Autodesk Fusion 360 part; units mm, degrees
(part 3 of 3)
sketch "bottom_d_plate" plane through (0, 0, 0) normal (0, 1, 0) x (1, 0, 0)
  arc A0 (69.1916, -25.8629) -> (70.1916, -26.8607) centre (70.1916, -25.8607) ccw
  line L0 (69.6545, -38.7668) -> (79.5366, -38.7668)
  circle A1 centre (53.7342, -72.0705) radius 1.7
  arc A2 (-18.6223, 40.5765) -> (-23.9656, 38.9319) centre (-18.6231, 31.0765) ccw
  line L1 (-55.4675, 17.5074) -> (-23.9656, 38.9319)
  arc A3 (53.2919, -80.5601) -> (61.3893, -75.8117) centre (53.1625, -71.0609) ccw
  line L2 (20.548, 40.3463) -> (46.7337, 34.5163)
  line L3 (69.0702, 28.465) -> (69.0699, 28.4264)
  arc A4 (80.543, 19.3715) -> (73.1075, 28.6444) centre (71.043, 19.3715) ccw
  line L4 (25.063, -80.0083) -> (-19.071, -59.5488)
  arc A5 (25.063, -80.0083) -> (29.1879, -80.8885) centre (29.0585, -71.3894) ccw
  line L5 (53.2919, -80.5601) -> (29.1879, -80.8885)
  line L6 (79.2698, -44.8485) -> (61.3893, -75.8117)
  arc A6 (79.2698, -44.8485) -> (80.5358, -39.7279) centre (71.043, -40.0977) ccw
  arc A7 (50.4596, -69.0135) -> (51.8256, -68.6475) centre (50.9596, -68.1475) ccw
  line L7 (-18.6223, 40.5765) -> (18.4843, 40.5734)
  circle A8 centre (-51.125, -50.075) radius 1.7
  circle A9 centre (72.1849, -22.8607) radius 1.7
  arc A10 (20.548, 40.3463) -> (18.4843, 40.5734) centre (18.4835, 31.0734) ccw
  line L8 (-50.125, -58.575) -> (-23.4871, -58.575)
  arc A11 (-59.625, -49.075) -> (-50.125, -58.575) centre (-50.125, -49.075) ccw
  line L9 (69.1916, -25.8629) -> (69.0702, 28.465)
  line L10 (80.543, 19.3715) -> (80.543, -25.8607)
  line L11 (73.1075, 28.6444) -> (70.2865, 29.3961)
  line L12 (-59.625, -49.075) -> (-59.625, 9.652)
  line L13 (69.0702, 28.465) -> (69.1309, 1.3011)
  arc A12 (70.3273, 29.3852) -> (69.0699, 28.4264) centre (70.0698, 28.4189) ccw
  arc A13 (-19.071, -59.5488) -> (-23.4871, -58.575) centre (-23.4871, -69.075) ccw
  circle A14 centre (72.1849, 20.1393) radius 1.7
  line L14 (70.2865, 29.3961) -> (70.3273, 29.3852)
  line L15 (46.7337, 34.5163) -> (46.8423, 34.4921)
  arc A15 (-55.4675, 17.5074) -> (-59.625, 9.652) centre (-50.125, 9.652) ccw
  circle A16 centre (-51.125, 10.1813) radius 1.7
  line L16 (80.543, -40.0977) -> (80.543, -39.4973)
  line L17 (70.1916, -26.8607) -> (79.543, -26.8607)
  arc A17 (80.5358, -39.7279) -> (79.5366, -38.7668) centre (79.5366, -39.7668) ccw
  arc A18 (79.543, -26.8607) -> (80.543, -25.8607) centre (79.543, -25.8607) ccw
  arc A19 (52.2962, -60.5122) -> (53.6622, -60.1462) centre (52.7962, -59.6462) ccw
  line L18 (13.286, -51.6) -> (1.286, -51.6)
  line L19 (36.0873, -42.1814) -> (24.4962, -39.0756)
  line L20 (33.6886, -54.9973) -> (36.7944, -43.4062)
  line L21 (45.1, -3) -> (45.1, -15)
  arc A20 (44.1, 17.05) -> (45.1, 16.05) centre (44.1, 16.05) cw
  circle A21 centre (-18.9309, 32.0765) radius 1.7
  line L22 (45.1, 16.05) -> (45.1, 4.05)
  line L23 (-32.1, 8.05) -> (-44.1, 8.05)
  arc A22 (-26.05, 19.05) -> (-25.05, 20.05) centre (-25.05, 19.05) cw
  line L24 (-12.05, -19.06) -> (-12.05, -31.06)
  circle A23 centre (43.1794, 26.5995) radius 1.7
  line L25 (7, 25.05) -> (7, 13.05)
  arc A24 (-31.1, 7.05) -> (-32.1, 8.05) centre (-32.1, 7.05) ccw
  line L26 (13.05, 0.5) -> (25.05, 0.5)
  arc A25 (6, 26.05) -> (7, 25.05) centre (6, 25.05) cw
  line L27 (6, 12.05) -> (-6, 12.05)
  line L28 (-44.1, -5.95) -> (-32.1, -5.95)
  line L29 (-32.1, -44.05) -> (-44.1, -44.05)
  arc A26 (-45.1, -31.05) -> (-44.1, -30.05) centre (-44.1, -31.05) cw
  line L30 (26.05, 18.55) -> (26.05, 6.55)
  arc A27 (-7, 6) -> (-6, 7) centre (-6, 6) cw
  line L31 (-31.1, -31.05) -> (-31.1, -43.05)
  arc A28 (6, 7) -> (7, 6) centre (6, 6) cw
  arc A29 (26.05, -12.5) -> (25.05, -13.5) centre (25.05, -12.5) cw
  arc A30 (-12.05, -31.06) -> (-13.05, -32.06) centre (-13.05, -31.06) cw
  circle A31 centre (-18.212, -50.5781) radius 1.7
  line L32 (-32.1, -25) -> (-44.1, -25)
  arc A32 (-12.05, -12) -> (-13.05, -13) centre (-13.05, -12) cw
  line L33 (-7, 13.05) -> (-7, 25.05)
  arc A33 (-45.1, -4.95) -> (-44.1, -5.95) centre (-44.1, -4.95) ccw
  line L34 (-7, -25.05) -> (-7, -13.05)
  line L35 (-25.05, -18.06) -> (-13.05, -18.06)
  arc A34 (-26.05, -19.06) -> (-25.05, -18.06) centre (-25.05, -19.06) cw
  line L36 (-44.1, -11) -> (-32.1, -11)
  arc A35 (6, -12.05) -> (7, -13.05) centre (6, -13.05) cw
  arc A36 (-45.1, -12) -> (-44.1, -11) centre (-44.1, -12) cw
  arc A37 (7, -25.05) -> (6, -26.05) centre (6, -25.05) cw
  line L37 (-45.1, -24) -> (-45.1, -12)
  line L38 (-26.05, 7.05) -> (-26.05, 19.05)
  arc A38 (32.1, 3.05) -> (31.1, 4.05) centre (32.1, 4.05) cw
  arc A39 (-13.05, -18.06) -> (-12.05, -19.06) centre (-13.05, -19.06) cw
  line L39 (32.1, 17.05) -> (44.1, 17.05)
  arc A40 (-13.05, 1) -> (-12.05, 0) centre (-13.05, 0) cw
  arc A41 (26.05, 6.55) -> (25.05, 5.55) centre (25.05, 6.55) cw
  arc A42 (-6, -7) -> (-7, -6) centre (-6, -6) cw
  line L40 (-13.05, 6.05) -> (-25.05, 6.05)
  line L41 (-13.05, -32.06) -> (-25.05, -32.06)
  arc A43 (13.05, 5.55) -> (12.05, 6.55) centre (13.05, 6.55) cw
  line L42 (7, 6) -> (7, -6)
  line L43 (-45.1, 7.05) -> (-45.1, -4.95)
  line L44 (26.05, -0.5) -> (26.05, -12.5)
  line L45 (-6, 26.05) -> (6, 26.05)
  line L46 (-31.1, -4.95) -> (-31.1, 7.05)
  line L47 (13.05, -18.55) -> (25.05, -18.55)
  arc A44 (-25.05, 6.05) -> (-26.05, 7.05) centre (-25.05, 7.05) cw
  arc A45 (-13.05, 20.05) -> (-12.05, 19.05) centre (-13.05, 19.05) cw
  arc A46 (-6, -26.05) -> (-7, -25.05) centre (-6, -25.05) cw
  arc A47 (-26.05, 0) -> (-25.05, 1) centre (-25.05, 0) cw
  arc A48 (-6, 12.05) -> (-7, 13.05) centre (-6, 13.05) cw
  line L48 (12.05, -12.5) -> (12.05, -0.5)
  arc A49 (12.05, -0.5) -> (13.05, 0.5) centre (13.05, -0.5) cw
  arc A50 (7, 13.05) -> (6, 12.05) centre (6, 13.05) cw
  arc A51 (-7, 25.05) -> (-6, 26.05) centre (-6, 25.05) cw
  arc A52 (-44.1, 8.05) -> (-45.1, 7.05) centre (-44.1, 7.05) ccw
  line L49 (7, -13.05) -> (7, -25.05)
  arc A53 (-32.1, -5.95) -> (-31.1, -4.95) centre (-32.1, -4.95) ccw
  arc A54 (12.05, -19.55) -> (13.05, -18.55) centre (13.05, -19.55) cw
  arc A55 (-32.1, -30.05) -> (-31.1, -31.05) centre (-32.1, -31.05) cw
  arc A56 (0.286, -38.6) -> (1.286, -37.6) centre (1.286, -38.6) cw
  circle A57 centre (18.5935, 32.0734) radius 1.7
  line L50 (6, -7) -> (-6, -7)
  arc A58 (-31.1, -43.05) -> (-32.1, -44.05) centre (-32.1, -43.05) cw
  arc A59 (-31.1, -24) -> (-32.1, -25) centre (-32.1, -24) cw
  line L51 (-31.1, -12) -> (-31.1, -24)
  line L52 (-45.1, -43.05) -> (-45.1, -31.05)
  arc A60 (1.286, -51.6) -> (0.286, -50.6) centre (1.286, -50.6) cw
  line L53 (0.286, -50.6) -> (0.286, -38.6)
  arc A61 (25.05, -18.55) -> (26.05, -19.55) centre (25.05, -19.55) cw
  arc A62 (-44.1, -25) -> (-45.1, -24) centre (-44.1, -24) cw
  line L54 (6, -26.05) -> (-6, -26.05)
  circle A63 centre (-51.125, -50.075) radius 1.7
  line L55 (-6, -12.05) -> (6, -12.05)
  arc A64 (-32.1, -11) -> (-31.1, -12) centre (-32.1, -12) cw
  line L56 (25.05, 5.55) -> (13.05, 5.55)
  line L57 (12.05, 6.55) -> (12.05, 18.55)
  line L58 (-6, 7) -> (6, 7)
  line L59 (13.05, 19.55) -> (25.05, 19.55)
  line L60 (-7, -6) -> (-7, 6)
  arc A65 (-44.1, -44.05) -> (-45.1, -43.05) centre (-44.1, -43.05) cw
  line L61 (-26.05, -31.06) -> (-26.05, -19.06)
  arc A66 (-7, -13.05) -> (-6, -12.05) centre (-6, -13.05) cw
  arc A67 (45.1, 4.05) -> (44.1, 3.05) centre (44.1, 4.05) cw
  arc A68 (25.05, 19.55) -> (26.05, 18.55) centre (25.05, 18.55) cw
  arc A69 (31.1, 16.05) -> (32.1, 17.05) centre (32.1, 16.05) cw
  arc A70 (7, -6) -> (6, -7) centre (6, -6) cw
  arc A71 (-25.05, -13) -> (-26.05, -12) centre (-25.05, -12) cw
  line L62 (-44.1, -30.05) -> (-32.1, -30.05)
  arc A72 (-25.05, -32.06) -> (-26.05, -31.06) centre (-25.05, -31.06) cw
  arc A73 (-12.05, 7.05) -> (-13.05, 6.05) centre (-13.05, 7.05) cw
  line L63 (-12.05, 19.05) -> (-12.05, 7.05)
  line L64 (25.05, -13.5) -> (13.05, -13.5)
  line L65 (-12.05, 0) -> (-12.05, -12)
  line L66 (-25.05, 20.05) -> (-13.05, 20.05)
  line L67 (44.1, 3.05) -> (32.1, 3.05)
  line L68 (31.1, 4.05) -> (31.1, 16.05)
  arc A74 (13.05, -13.5) -> (12.05, -12.5) centre (13.05, -12.5) cw
  line L69 (-13.05, -13) -> (-25.05, -13)
  arc A75 (12.05, 18.55) -> (13.05, 19.55) centre (13.05, 18.55) cw
  line L70 (-25.05, 1) -> (-13.05, 1)
  line L71 (31.1, -15) -> (31.1, -3)
  line L72 (32.1, -2) -> (44.1, -2)
  line L73 (1.286, -37.6) -> (13.286, -37.6)
  line L74 (32.1, -21.05) -> (44.1, -21.05)
  arc A76 (13.05, -32.55) -> (12.05, -31.55) centre (13.05, -31.55) cw
  line L75 (23.2714, -39.7827) -> (20.1656, -51.3738)
  arc A77 (57.1204, -38.6328) -> (57.6205, -38.7668) centre (57.6205, -37.7668) ccw
  arc A78 (44.1, -21.05) -> (45.1, -22.05) centre (44.1, -22.05) cw
  line L76 (26.05, -19.55) -> (26.05, -31.55)
  line L77 (47.625, 33.516) -> (47.625, -32.5721)
  line L78 (-26.05, -12) -> (-26.05, 0)
  line L79 (31.1, -34.05) -> (31.1, -22.05)
  line L80 (45.1, -22.05) -> (45.1, -34.05)
  line L81 (12.05, -31.55) -> (12.05, -19.55)
  arc A79 (25.05, 0.5) -> (26.05, -0.5) centre (25.05, -0.5) cw
  arc A80 (59.6622, -49.7538) -> (59.2962, -48.3878) centre (58.7962, -49.2538) ccw
  line L82 (59.2962, -48.3878) -> (48.9038, -42.3878)
  arc A81 (48.9038, -42.3878) -> (47.5378, -42.7538) centre (48.4038, -43.2538) ccw
  arc A82 (20.1656, -51.3738) -> (20.8727, -52.5986) centre (21.1315, -51.6326) ccw
  line L83 (20.8727, -52.5986) -> (32.4638, -55.7044)
  line L84 (44.1, -35.05) -> (32.1, -35.05)
  arc A83 (32.4638, -55.7044) -> (33.6886, -54.9973) centre (32.7226, -54.7385) ccw
  line L85 (14.286, -38.6) -> (14.286, -50.6)
  line L86 (48.1249, -33.4381) -> (57.1204, -38.6328)
  line L87 (25.05, -32.55) -> (13.05, -32.55)
  circle A84 centre (71.1231, -41.9588) radius 1.7
  arc A85 (41.5378, -53.1462) -> (41.9038, -54.5122) centre (42.4038, -53.6462) ccw
  arc A86 (14.286, -50.6) -> (13.286, -51.6) centre (13.286, -50.6) cw
  line L88 (53.6622, -60.1462) -> (59.6622, -49.7538)
  circle A87 centre (28.4977, -72.2317) radius 1.7
  arc A88 (36.7944, -43.4062) -> (36.0873, -42.1814) centre (35.8285, -43.1474) ccw
  line L89 (41.9038, -54.5122) -> (52.2962, -60.5122)
  arc A89 (45.1, -34.05) -> (44.1, -35.05) centre (44.1, -34.05) cw
  arc A90 (47.625, -32.5721) -> (48.1249, -33.4381) centre (48.625, -32.5721) ccw
  arc A91 (24.4962, -39.0756) -> (23.2714, -39.7827) centre (24.2374, -40.0415) ccw
  arc A92 (13.286, -37.6) -> (14.286, -38.6) centre (13.286, -38.6) cw
  line L90 (47.5378, -42.7538) -> (41.5378, -53.1462)
  arc A93 (44.1, -2) -> (45.1, -3) centre (44.1, -3) cw
  arc A94 (31.1, -22.05) -> (32.1, -21.05) centre (32.1, -22.05) cw
  arc A95 (31.1, -3) -> (32.1, -2) centre (32.1, -3) cw
  arc A96 (32.1, -35.05) -> (31.1, -34.05) centre (32.1, -34.05) cw
  arc A97 (45.1, -15) -> (44.1, -16) centre (44.1, -15) cw
  line L91 (44.1, -16) -> (32.1, -16)
  arc A98 (26.05, -31.55) -> (25.05, -32.55) centre (25.05, -31.55) cw
  arc A99 (32.1, -16) -> (31.1, -15) centre (32.1, -15) cw
  arc A100 (47.625, 33.516) -> (46.8423, 34.4921) centre (46.625, 33.516) ccw
  line L92 (69.6545, -38.7668) -> (57.6205, -38.7668)
  dimension "d158" = 1
  dimension "d160" = 1
  dimension "d161" = 1
  dimension "d162" = 1
  constraint tangent A6 L16
  constraint perpendicular L0 L16
  constraint tangent L0 A17
  constraint tangent A6 A17
  constraint parallel L2 L15
  constraint parallel L9 L13
  constraint parallel L11 L14
  constraint tangent L3 A12
  constraint tangent A12 L14
  constraint tangent L15 A100
  constraint tangent L77 A100
  constraint tangent A77 L92
  measures "d158" radius of A17
  measures "d160" radius of A12
  measures "d161" radius of A7
  measures "d162" radius of A100
equation "wall_thickness = 2 mm"
equation "plate_tab_depth = 4 mm"
equation "pcb_clearance = 1 mm"
equation "tolerance = 0.4 mm"
equation "m2_standoff = 3.4 mm"
equation "m2_screwhole = 2.2 mm"
equation "border_width = 8 mm"
equation "d42 = border_curve_allowance + border_width"
equation "d43 = border_width + border_curve_allowance"
equation "d44 = border_width + border_curve_allowance"
equation "d45 = border_width + border_curve_allowance"
equation "d46 = border_width + border_curve_allowance"
equation "d48 = border_width + border_curve_allowance"
equation "d53 = border_width + border_curve_allowance"
equation "border_curve_allowance = 4.5 mm"
equation "d59 = m2_standoff"
equation "d62 = m2_screwhole"
equation "d63 = m2_standoff"
equation "d64 = m2_screwhole"
equation "d65 = m2_standoff"
equation "d66 = m2_screwhole"
equation "d68 = m2_standoff"
equation "d69 = m2_screwhole"
equation "d72 = bevel_depth"
equation "d73 = m2_standoff"
equation "d74 = m2_screwhole"
equation "d75 = m2_standoff"
equation "d76 = m2_screwhole"
equation "d78 = m2_standoff"
equation "d79 = m2_screwhole"
equation "d80 = bevel_depth"
equation "d81 = bevel_depth"
equation "d82 = m2_standoff"
equation "d83 = m2_screwhole"
equation "d84 = bevel_depth"
equation "d85 = bevel_depth"
equation "d86 = m2_standoff"
equation "d87 = m2_screwhole"
equation "d88 = bevel_depth"
equation "d89 = bevel_depth"
equation "d90 = m2_standoff"
equation "d91 = m2_screwhole"
equation "d92 = m2_standoff"
equation "d93 = m2_screwhole"
equation "d94 = bevel_depth"
equation "bevel_depth = 9 mm"
equation "d100 = bevel_depth"
equation "d101 = bevel_depth"
equation "d102 = bevel_depth"
equation "d103 = bevel_depth"
equation "d104 = bevel_depth"
equation "d105 = bevel_depth"
equation "stepA = 0.5 mm"
equation "stepB = 1.75 mm"
equation "stepC = 5.5 mm"
equation "d117 = -plate_thickness"
equation "plate_thickness = 1.6 mm"
equation "d129 = -stepA"
equation "d130 = stepB"
equation "d131 = stepC"
named bodies: "plate_main", "plate_second"
